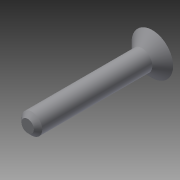
# Autodesk Inventor part: DIN7991x30
Saved by Autodesk Inventor 2013 (Build 170138000, 138)
## iProperties
Created: 2015-01-15
Part Number: DIN7991x30
Material: Generic
Document SubType Name: Modeling
Designer: dzban
Density: 1 g/cm^3
Author: dzban
Autodesk Inventor part; units mm, degrees
ref_plane "YZ Plane" through (0, 0, 0) normal (1, 0, 0) x (0, 1, 0)
ref_plane "XZ Plane" through (0, 0, 0) normal (0, 1, 0) x (-1, 0, 0)
ref_plane "XY Plane" through (0, 0, 0) normal (0, 0, 1) x (1, 0, 0)
sketch "Sketch1" plane through (0, 0, 0) normal (0, 0, 1) x (1, 0, 0)
  line L0 (0, 0) -> (0, 30)
  line L1 (0, 30) -> (5, 30)
  line L2 (5, 30) -> (2.5, 27.5)
  line L3 (2.5, 27.5) -> (2.5, 1)
  line L4 (1.5, 0) -> (0, 0)
  line L5 (2.5, 1) -> (1.5, 0)
  point P0 (2.5, 0)
  dimension "d0" = 2.5
  dimension "d2" = 5
  dimension "d3" = 135
  dimension "d4" = 30
  dimension "d6" = 1
  dimension "d7" = 1
  constraints: 12 end point, 2 horizontal, 2 point on line, 2 vertical
  measures "d0" distance between parallel lines of L3 L0
  measures "d2" distance from line of L1.end L0
  measures "d3" angle of L2 L3
  measures "d4" distance between parallel lines of L1 L4
  measures "d6" distance of L3.end point (2.5, 0)
  measures "d7" distance of L4.start point (2.5, 0)
revolve "Revolution1" add sketch "Sketch1" angle 360 about axis through (0, 0, 0) along (0, 1, 0)
sketch "Sketch2" plane through (0, 30, 0) normal (0, 1, 0) x (1, 0, 0)
  circle A0 centre (0, 0) radius 5 projected
  line L0 (1.4802, -0.8994) -> (-0.0388, -1.7316)
  line L1 (-0.0388, -1.7316) -> (-1.519, -0.8322)
  line L2 (-1.519, -0.8322) -> (-1.4802, 0.8994)
  line L3 (-1.4802, 0.8994) -> (0.0388, 1.7316)
  line L4 (0.0388, 1.7316) -> (1.519, 0.8322)
  line L5 (1.519, 0.8322) -> (1.4802, -0.8994)
  dimension "d8" = 3
  constraints: 12 end point, 1 coincident, 13 other
  measures "d8" distance between parallel lines of L3 L0
extrude "Extrusion1" cut sketch "Sketch2" against normal blind 2 contours L0 L1 L2 L3 L4 L5
equation "\"d7\" = d6"
body "Solid1"
